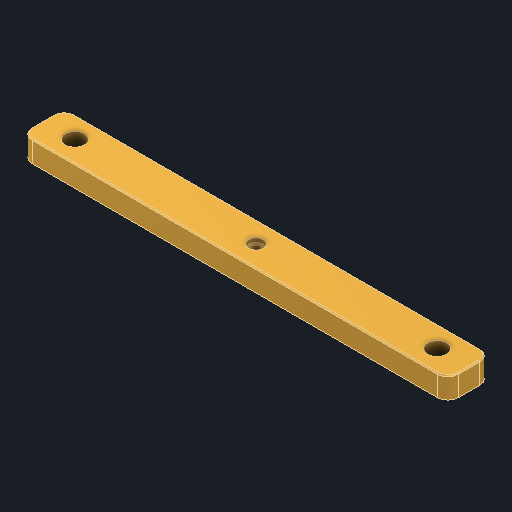
# Autodesk Inventor part: Lower Arm Brass Plate
Saved by Autodesk Inventor 2027.1 (Build 311270010, 270A)
## iProperties
Created: 2025-09-16
Material: Brass, Soft Yellow
Document SubType Name: Modeling
Designer: SD
Density: 8.47 g/cm^3
Appearance: Brass - Satin
Mass: 326.52 g
Surface Area: 128.304 cm^2
Volume: 38.5502 cm^3
Project: Automatic Tea Steeping mechanism
Part Number: Lower Arm Brass Plate
Length: 200.000 mm
Width: 20.000 mm
Thickness: 10.000 mm
BOM-Mass: 0.32652
BOM-Area: 0.013
Procurement: Fabricate - 1st round
Build Stage: 1
Preferred Material: C36000 Brass
Author: SD
Title: Lower Arm Brass Plate
Autodesk Inventor part; units mm, degrees
ref_plane "YZ Plane" through (0, 0, 0) normal (1, 0, 0) x (0, 1, 0)
ref_plane "XZ Plane" through (0, 0, 0) normal (0, 1, 0) x (-1, 0, 0)
ref_plane "XY Plane" through (0, 0, 0) normal (0, 0, 1) x (1, 0, 0)
sketch "Sketch1" plane through (0, 0, 0) normal (0, 1, 0) x (-1, 0, 0)
  line L0 (-100, 10) -> (100, 10)
  line L1 (100, 10) -> (100, -10)
  line L2 (100, -10) -> (-100, -10)
  line L3 (-100, -10) -> (-100, 10)
  line L4 (-100, 10) -> (100, -10) construction
  line L5 (100, 10) -> (-100, -10) construction
  point P0 (0, 0)
  dimension "Length" = 200
  dimension "Width" = 20
  constraints: 12 end point, 2 midpoint, 2 parallel, 1 horizontal, 1 perpendicular
  measures "Length" distance of L1.end L2.end
  measures "Width" distance of L0.end L1.end
extrude "Extrusion1" add sketch "Sketch1" along normal mid plane 10
sketch "Sketch2" plane through (0, 5, 0) normal (0, 1, 0) x (1, 0, 0)
  circle A0 centre (0, 0) radius 2
  dimension "d4" = 4
  constraints: 1 centre point, 1 coincident
  measures "d4" diameter of A0
extrude "Extrusion2" cut sketch "Sketch2" against normal up to surface (10 mm away)
sketch "Sketch3" plane through (0, 5, 0) normal (0, 1, 0) x (1, 0, 0)
  circle A0 centre (0, 0) radius 2 projected
  point P0 (-15, 0)
  point P1 (15, 0)
  dimension "d7" = 30
  dimension "d8" = 15
  constraints: 2 horizontal alignment
  measures "d7" distance of point (15, 0) point (-15, 0)
  measures "d8" distance of A0.centre point (15, 0)
hole "Hole1" [suppressed]
sketch "Sketch4" plane through (0, 5, 0) normal (0, 1, 0) x (1, 0, 0)
  point P0 (0, 0)
  point P1 (-85, 0)
  point P2 (85, 0)
  dimension "d16" = 170
  dimension "d17" = 85
  constraints: 2 horizontal alignment
  measures "d16" distance of point (85, 0) point (-85, 0)
  measures "d17" distance of point (0, 0) point (85, 0)
hole "Hole2" at (-85, 5, 0) at (85, 5, 0) direction (0, -1, 0) diameter 9 end through all
sketch "Sketch5" plane through (0, 5, 0) normal (0, 1, 0) x (1, 0, 0)
  circle A0 centre (0, 0) radius 2 projected
  circle A1 centre (0, 0) radius 3.5
  dimension "d25" = 7
  constraints: 1 centre point, 1 coincident
  measures "d25" diameter of A1
extrude "Extrusion3" cut sketch "Sketch5" against normal blind 2
fillet "Fillet1" radius 5 4 edges at (-100, 0, 10) (-100, 0, -10) (100, 0, 10) (100, 0, -10)
chamfer "Chamfer1" distance 0.5 angle 45 8 edges at (0, 5, 10) (98.5355, 5, 8.5355) (100, 5, 0) (98.5355, 5, -8.5355) (0, 5, -10) (-98.5355, 5, -8.5355) (-100, 5, 0) (-98.5355, 5, 8.5355)
equation "\"d8\" = 0.5 * d7"
equation "\"d17\" = 0.5 * d16"
body "Solid1"
